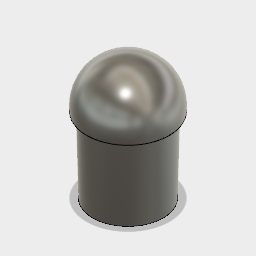
Bike Handle Plug (f360) (Autodesk Fusion 360 design; units mm, degrees)
Autodesk Fusion 360 part; units mm, degrees
sketch "Sketch1" plane through (0, 0, 0) normal (0, 1, 0) x (1, 0, 0) in component "Component"
  line L0 (25.4068, -5.2075) -> (44.4514, -5.6403)
  line L1 (25.4068, -5.2075) -> (25.4068, -4.0649)
  line L2 (13.6241, -14.6055) -> (44.4514, -14.6055)
  arc A0 (25.4068, -4.0649) -> (13.6241, -14.6055) centre (24.0027, -14.3512) ccw
  line L3 (44.4514, -5.6403) -> (44.4514, -14.6055)
  dimension "d11" = 9.398
  measures "d11" distance of L0.start L2
revolve "Revolve1" add sketch "Sketch1" angle 360 about axis through (13.6241, 0, 14.6055) along (1, 0, 0) in component "Component"
move_body "Move1" bodies 1 to x (0, -1, 0) y (1, 0, 0) z (0, 0, 1) at (24.0025, 2.736, 0) in component "Component"
component "Component" placed x (1, 0, 0) y (0, 1, 0) z (0, 0, 1) at (0, 0, 0)
